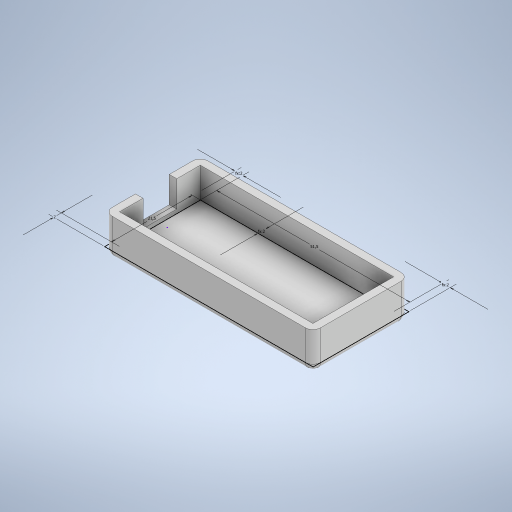
# Autodesk Inventor part: case pico
Saved by Autodesk Inventor 2024 (Build 280153000, 153)
## iProperties
Created: 2024-03-01
Part Number: case pico
Material: Generic
Document SubType Name: Modeling
Designer: quinten
Density: 1 g/cm^3
Appearance: Default
Author: quinten
Autodesk Inventor part; units mm, degrees
ref_plane "YZ Plane" through (0, 0, 0) normal (1, 0, 0) x (0, 1, 0)
ref_plane "XZ Plane" through (0, 0, 0) normal (0, 1, 0) x (-1, 0, 0)
ref_plane "XY Plane" through (0, 0, 0) normal (0, 0, 1) x (1, 0, 0)
sketch "Sketch1" plane through (0, 0, 0) normal (0, 1, 0) x (-1, 0, 0)
  line L0 (0, 0) -> (51.5, 0)
  line L1 (51.5, 0) -> (51.5, -21.5)
  line L2 (51.5, -21.5) -> (0, -21.5)
  line L3 (0, -21.5) -> (0, 0)
  line L4 (53.5, 2) -> (-2, 2)
  line L5 (-2, 2) -> (-2, -23.5)
  line L6 (-2, -23.5) -> (53.5, -23.5)
  line L7 (53.5, -23.5) -> (53.5, 2)
  point P0 (49.5, -10.75)
  dimension "d0" = 51.5
  dimension "d1" = 21.5
  dimension "d2" = 2
  dimension "d3" = 2
  dimension "d4" = 2
  dimension "d5" = 2
  constraints: 16 end point, 4 parallel, 2 horizontal, 2 perpendicular
  measures "d0" distance of L1.end L2.end
  measures "d1" distance of L0.end L1.end
  measures "d2" distance between parallel lines of L6 L2
  measures "d3" distance between parallel lines of L7 L1
  measures "d4" distance between parallel lines of L0 L4
  measures "d5" distance between parallel lines of L3 L5
extrude "Extrusion2" add sketch "Sketch1" against normal blind 2 contours L0 L1 L2 L3 | L7 L6 L5 L4
extrude "Extrusion3" add sketch "Sketch1" along normal blind 8
sketch "Sketch2" plane through (0, 8, 0) normal (0, 1, 0) x (1, 0, 0)
  line L0 (-51.5, 6.25) -> (-51.5, 15.25) construction
  line L1 (-51.5, 0) -> (-51.5, 21.5) projected
  line L2 (-51.5, 6.25) -> (-53.5, 6.25)
  line L3 (-53.5, -2) -> (-53.5, 23.5) projected
  line L4 (-51.5, 15.25) -> (-53.5, 15.25)
  point P0 (0, 0)
  point P1 (-51.5, 10.75)
  dimension "d20" = 9
  constraints: 6 end point, 2 midpoint, 2 point on line, 1 horizontal, 1 parallel, 1 vertical
  measures "d20" distance of L0.start L0.end
extrude "Extrusion4" cut sketch "Sketch2" against normal blind 7
fillet "Fillet1" radius 2 8 edges at (2, 3, 2) (2, 3, -23.5) (-53.5, 3, 2) (-53.5, 3, -23.5) (-53.5, -2, -10.75) (-25.75, -2, -23.5) (2, -2, -10.75) (-25.75, -2, 2)
equation "\"d2\" = d4"
equation "\"d3\" = d4"
equation "\"d5\" = d4"
body "Solid1"
